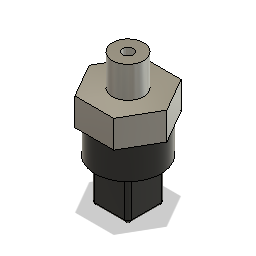
Logger_V1 v25 (Autodesk Fusion 360 archive; units mm, degrees)
design "圧力センサ"
Autodesk Fusion 360 part; units mm, degrees
sketch "スケッチ1" plane through (0, 0, 0) normal (0, 1, 0) x (1, 0, 0)
  line L0 (0, 11) -> (-6.3509, 11)
  line L1 (0, 0) -> (11, 0) construction
  line L2 (-9.5263, 5.5) -> (-6.3509, 11)
  line L3 (-9.5263, 5.5) -> (-3.1754, 5.5) construction
  line L4 (-9.5263, -5.5) -> (-12.7017, 0)
  line L5 (-9.5263, 5.5) -> (-12.7017, 0)
  line L6 (0, -11) -> (-6.3509, -11)
  line L7 (-9.5263, -5.5) -> (-6.3509, -11)
  line L8 (9.5263, -5.5) -> (6.3509, -11)
  line L9 (0, -11) -> (6.3509, -11)
  line L10 (9.5263, 5.5) -> (12.7017, 0)
  line L11 (9.5263, -5.5) -> (12.7017, 0)
  line L12 (0, 11) -> (6.3509, 11)
  line L13 (9.5263, 5.5) -> (6.3509, 11)
  circle A0 centre (0, 0) radius 5.1
  dimension "d1" = 11
  dimension "d3" = 11
  dimension "d4" = 60
  dimension "d6" = 360
  dimension "d7" = 10.2
  constraint horizontal L1
  constraint coincident L1.start A0.centre
  constraint horizontal L3
  measures "d1" distance of L1.start L0.start
  measures "d3" distance of L1.start L2.start
  measures "d4" angle of L2 L3
  measures "d7" diameter of A0
extrude "押し出し1" add sketch "スケッチ1" along normal blind 9 makes body 1
extrude "押し出し2" add sketch "スケッチ1" along normal blind 19.2 contours A0 bodies 1
sketch "スケッチ2" plane through (0, 19.2, 0) normal (0, 1, 0) x (-1, 0, 0)
  circle A0 centre (0, 0) radius 5.1
  circle A1 centre (0, 0) radius 1.75
  dimension "d12" = 3.5
  constraint coincident A0.centre A1.centre
  measures "d12" diameter of A1
extrude "押し出し3" cut sketch "スケッチ2" against normal blind 10 contours A1 bodies 1
sketch "スケッチ3" plane through (0, 0, 0) normal (0, -1, 0) x (1, 0, 0)
  line L0 (12.7017, 0) -> (6.3509, 11)
  line L1 (6.3509, 11) -> (-6.3509, 11)
  line L2 (-6.3509, 11) -> (-12.7017, 0)
  line L3 (-12.7017, 0) -> (-6.3509, -11)
  line L4 (-6.3509, -11) -> (6.3509, -11)
  line L5 (6.3509, -11) -> (12.7017, 0)
  circle A0 centre (0, 0) radius 10.75
  dimension "d15" = 21.5
  constraint coincident A0.centre origin
  measures "d15" diameter of A0
extrude "押し出し4" add sketch "スケッチ3" along normal blind 10 separate body contours A0 makes body 2
sketch "スケッチ4" plane through (0, -10, 0) normal (0, -1, 0) x (1, 0, 0)
  circle A0 centre (0, 0) radius 10.75
  line L0 (6, 6) -> (-6, 6)
  line L1 (-6, 6) -> (-6, -6)
  line L2 (-6, -6) -> (6, -6)
  line L3 (6, -6) -> (6, 6)
  line L4 (6, 6) -> (-6, -6) construction
  line L5 (-6, 6) -> (6, -6) construction
  dimension "d18" = 12
  dimension "d19" = 12
  constraint horizontal L0
  constraint perpendicular L0 L1
  constraint parallel L0 L2
  constraint parallel L1 L3
  constraint coincident L4 A0.centre
  constraint coincident L5 A0.centre
  constraint coincident A0.centre origin
  measures "d18" distance of L1.end L2.end
  measures "d19" distance of L0.end L1.end
extrude "押し出し5" add sketch "スケッチ4" along normal blind 14 contours L0 L1 L2 L3 bodies 2
fillet "フィレット1" radius 1 4 edges at (6, -17, -6) (6, -17, 6) (-6, -17, 6) (-6, -17, -6) on bodies 2
fillet "フィレット2" radius 1 8 edges at (5.7071, -24, -5.7071) (6, -24, 0) (5.7071, -24, 5.7071) (0, -24, 6) (-5.7071, -24, 5.7071) (-6, -24, 0) (-5.7071, -24, -5.7071) (0, -24, -6) on bodies 2
